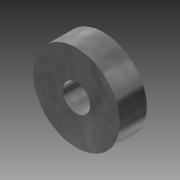
# Autodesk Inventor part: 625ZZ
Saved by Autodesk Inventor 2013 (Build 170138000, 138)
## iProperties
Created: 2014-06-28
Part Number: 625ZZ
Material: Generic
Document SubType Name: Modeling
Designer: Masta
Density: 1 g/cm^3
Author: Masta
Autodesk Inventor part; units mm, degrees
ref_plane "YZ Plane" through (0, 0, 0) normal (1, 0, 0) x (0, 1, 0)
ref_plane "XZ Plane" through (0, 0, 0) normal (0, 1, 0) x (-1, 0, 0)
ref_plane "XY Plane" through (0, 0, 0) normal (0, 0, 1) x (1, 0, 0)
sketch "Sketch1" plane through (0, 0, 0) normal (0, 1, 0) x (-1, 0, 0)
  circle A0 centre (0, 0) radius 2.5
  circle A1 centre (0, 0) radius 8
  dimension "d0" = 5
  dimension "d1" = 16
  constraints: 2 centre point, 2 coincident
  measures "d0" diameter of A0
  measures "d1" diameter of A1
extrude "Extrusion1" add sketch "Sketch1" along normal blind 5
body "Solid1"
